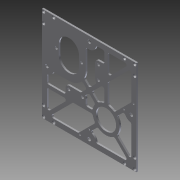
# Autodesk Inventor part: upper gearbox top plate2
Saved by Autodesk Inventor 2012 (Build 160160000, 160)
## iProperties
Created: 2012-07-07
Part Number: upper gearbox top plate2
Material: Default
Document SubType Name: Modeling
Designer: Bryce
Density: 1 g/cm^3
Author: Bryce
Autodesk Inventor part; units mm, degrees
ref_plane "YZ Plane" through (0, 0, 0) normal (1, 0, 0) x (0, 1, 0)
ref_plane "XZ Plane" through (0, 0, 0) normal (0, 1, 0) x (-1, 0, 0)
ref_plane "XY Plane" through (0, 0, 0) normal (0, 0, 1) x (1, 0, 0)
sketch "Sketch1" plane through (0, 0, 0) normal (0, 0, 1) x (1, 0, 0)
  line L0 (-114.3, 114.3) -> (63.5, 114.3)
  line L1 (63.5, 114.3) -> (63.5, -28.575)
  line L2 (63.5, -63.5) -> (28.575, -63.5)
  line L3 (-114.3, -63.5) -> (-114.3, 114.3)
  circle A0 centre (6.35, -6.35) radius 19.05
  circle A1 centre (41.275, 111.125) radius 1.5875
  circle A2 centre (-92.075, -60.325) radius 1.5875
  circle A3 centre (-111.125, 92.075) radius 1.5875
  circle A4 centre (-111.125, 111.125) radius 1.5875
  circle A5 centre (-92.075, 111.125) radius 1.5875
  circle A6 centre (60.325, 92.075) radius 1.5875
  circle A7 centre (-111.125, -60.325) radius 1.5875
  circle A8 centre (-111.125, -41.275) radius 1.5875
  circle A9 centre (60.325, 111.125) radius 1.5875
  circle A10 centre (-63.5, 73.025) radius 19.05
  circle A11 centre (-63.5, 53.975) radius 19.05
  line L4 (-82.55, 73.025) -> (-44.45, 73.025)
  line L5 (-44.45, 73.025) -> (-44.45, 53.975)
  line L6 (-44.45, 53.975) -> (-82.55, 53.975)
  line L7 (-82.55, 53.975) -> (-82.55, 73.025)
  arc A12 (-13.7147, 9.2246) -> (-18.8508, -3.175) centre (6.35, -6.35) ccw
  arc A13 (26.4147, -21.9246) -> (26.4147, 9.2246) centre (6.35, -6.35) ccw
  arc A14 (-9.2246, -26.4147) -> (21.9246, -26.4147) centre (6.35, -6.35) ccw
  arc A15 (21.9246, 13.7147) -> (9.525, 18.8508) centre (6.35, -6.35) ccw
  line L8 (-63.5, 14.3002) -> (-38.1, 14.3002)
  line L9 (-14.3002, 50.8) -> (-14.3002, 76.2)
  arc A16 (-63.3483, 22.2254) -> (-38.6735, 34.1834) centre (-63.5, 53.975) ccw
  line L10 (53.975, 104.775) -> (53.975, 45.7651)
  line L11 (53.975, -53.975) -> (49.4849, -53.975) construction
  line L12 (-104.775, -53.975) -> (-104.775, 12.7)
  line L13 (-63.3483, 22.2254) -> (-92.4782, 22.2254)
  line L14 (21.9246, -26.4147) -> (36.7849, -41.275)
  line L15 (26.4147, -21.9246) -> (41.275, -36.7849)
  line L16 (-13.7147, -21.9246) -> (-45.7651, -53.975)
  line L17 (-9.2246, -26.4147) -> (-24.1468, -41.337)
  line L18 (-13.7147, 9.2246) -> (-25.4, 20.9099)
  line L19 (-9.2246, 13.7147) -> (-20.9099, 25.4)
  line L20 (26.4147, 9.2246) -> (41.337, 24.1468)
  line L21 (21.9246, 13.7147) -> (53.975, 45.7651)
  arc A17 (-35.1635, 39.6536) -> (-31.75, 53.975) centre (-63.5, 53.975) ccw
  line L22 (53.975, -49.4849) -> (53.975, -53.975) construction
  line L23 (49.4849, -53.975) -> (36.7849, -53.975)
  line L24 (-45.7651, -53.975) -> (-104.775, -53.975)
  arc A18 (-31.75, 7.9502) -> (-33.7416, 12.5683) centre (-38.1, 7.9502) ccw
  line L25 (-104.775, -53.975) -> (-60.325, -9.525)
  line L26 (-104.775, -49.4849) -> (-64.8151, -9.525)
  line L27 (53.975, 104.775) -> (9.525, 60.325)
  line L28 (53.975, 100.2849) -> (9.525, 55.8349)
  line L29 (49.4849, 104.775) -> (9.525, 64.8151)
  line L30 (-40.9899, 14.3002) -> (-29.8901, 25.4)
  line L31 (-20.9099, 25.4) -> (-1.8599, 44.45)
  line L32 (-29.8901, 25.4) -> (-38.6735, 34.1834)
  line L33 (-25.4, 29.8901) -> (-35.1635, 39.6536)
  line L34 (-18.8508, -3.175) -> (-31.75, -3.175)
  line L35 (-104.775, -9.525) -> (-64.8151, -9.525)
  line L36 (-69.85, 7.9502) -> (-69.85, -3.175)
  line L37 (-31.75, 7.9502) -> (-31.75, -3.175)
  line L38 (-69.85, -3.175) -> (-104.775, -3.175)
  arc A19 (-31.75, 7.9502) -> (-33.7416, 12.5683) centre (-38.1, 7.9502) ccw
  arc A20 (-18.8508, -9.525) -> (-13.7147, -21.9246) centre (6.35, -6.35) ccw
  line L39 (-55.8349, -9.525) -> (-100.2849, -53.975)
  line L40 (9.525, 104.775) -> (9.525, 64.8151)
  line L41 (3.175, 104.775) -> (3.175, 82.55)
  arc A21 (3.175, 18.8508) -> (-9.2246, 13.7147) centre (6.35, -6.35) ccw
  line L42 (-7.9502, 82.55) -> (3.175, 82.55)
  line L43 (-7.9502, 44.45) -> (3.175, 44.45)
  line L44 (3.175, 44.45) -> (3.175, 18.8508)
  line L45 (-55.8349, -9.525) -> (-18.8508, -9.525)
  line L46 (9.525, 55.8349) -> (9.525, 18.8508)
  arc A22 (-33.7416, 12.5683) -> (-38.1, 14.3002) centre (-38.1, 7.9502) ccw
  arc A23 (-33.7416, 12.5683) -> (-38.1, 14.3002) centre (-38.1, 7.9502) ccw
  line L47 (-33.7416, 12.5683) -> (-25.4, 20.9099)
  arc A24 (-63.5, 14.3002) -> (-69.85, 7.9502) centre (-63.5, 7.9502) ccw
  line L48 (36.7849, -53.975) -> (-12.7, -53.975)
  line L49 (53.975, -36.7849) -> (53.975, -49.4849)
  line L50 (41.275, -36.7849) -> (53.975, -49.4849)
  line L51 (36.7849, -41.275) -> (49.4849, -53.975)
  line L52 (28.575, -63.5) -> (-114.3, -63.5)
  line L53 (63.5, -28.575) -> (63.5, -63.5)
  line L54 (-25.4, -53.975) -> (-25.4, -63.5) construction
  circle A25 centre (41.275, -60.325) radius 1.5875
  circle A26 centre (60.325, -60.325) radius 1.5875
  circle A27 centre (60.325, -41.275) radius 1.5875
  arc A28 (-7.9502, 82.55) -> (-14.3002, 76.2) centre (-7.9502, 76.2) ccw
  line L55 (6.35, -6.35) -> (-25.0809, -37.7809) construction
  line L56 (-43.0414, -55.7414) -> (-50.8, -63.5) construction
  line L57 (-25.0809, -37.7809) -> (-43.0414, -55.7414) construction
  line L58 (6.35, -6.35) -> (40.026, 27.326) construction
  line L59 (40.026, 27.326) -> (57.9865, 45.2865) construction
  line L60 (57.9865, 45.2865) -> (63.5, 50.8) construction
  arc A29 (-12.7, -53.975) -> (-24.1468, -41.337) centre (-25.4, -53.975) ccw
  arc A30 (41.337, 24.1468) -> (53.975, 12.7) centre (53.975, 25.4) ccw
  line L61 (53.975, 12.7) -> (53.975, -36.7849)
  arc A31 (-31.75, 93.7765) -> (-12.7, 104.775) centre (-25.4, 104.775) ccw
  line L62 (-31.75, 93.7765) -> (-31.75, 53.975)
  line L63 (-12.7, 104.775) -> (53.975, 104.775)
  arc A32 (-104.775, 12.7) -> (-92.4782, 22.2254) centre (-104.775, 25.4) ccw
  arc A33 (-14.3002, 50.8) -> (-7.9502, 44.45) centre (-7.9502, 50.8) ccw
  line L64 (-25.4, 29.8901) -> (-10.3636, 44.9265)
  point P0 (0, 0)
  point P1 (-87.3125, 63.5)
  point P2 (-39.6875, 63.5)
  point P3 (-38.1, 7.9502)
  dimension "d87" = 38.1
  dimension "d89" = 38.1
  dimension "d0" = 114.3
  dimension "d1" = 177.8
  dimension "d2" = 177.8
  dimension "d3" = 114.3
  dimension "d4" = 38.1
  dimension "d5" = 57.15
  dimension "d6" = 57.15
  dimension "d10" = 3.175
  dimension "d12" = 3.175
  dimension "d15" = 3.175
  dimension "d16" = 22.225
  dimension "d19" = 3.175
  dimension "d20" = 22.225
  dimension "d23" = 3.175
  dimension "d24" = 3.175
  dimension "d25" = 22.225
  dimension "d26" = 3.175
  dimension "d27" = 3.175
  dimension "d28" = 3.175
  dimension "d29" = 3.175
  dimension "d30" = 22.225
  dimension "d34" = 3.175
  dimension "d35" = 3.175
  dimension "d36" = 3.175
  dimension "d37" = 3.175
  dimension "d38" = 22.225
  dimension "d39" = 3.175
  dimension "d40" = 3.175
  dimension "d47" = 3.175
  dimension "d48" = 3.175
  dimension "d49" = 3.175
  dimension "d50" = 3.175
  dimension "d51" = 22.225
  dimension "d52" = 3.175
  dimension "d88" = 41.275
  dimension "d91" = 50.8
  dimension "d95" = 19.05
  dimension "d98" = 23.8125
  dimension "d99" = 23.8125
  dimension "d112" = 25.4
  dimension "d113" = 71.4502
  dimension "d114" = 50.8
  dimension "d122" = 71.4502
  dimension "d123" = 25.4
  dimension "d124" = 38.1
  dimension "d140" = 25.4
  dimension "d141" = 25.4
  dimension "d142" = 25.4
  dimension "d143" = 25.4
  dimension "d160" = 6.35
  dimension "d163" = 6.35
  dimension "d167" = 9.525
  dimension "d168" = 9.525
  dimension "d169" = 31.75
  dimension "d171" = 158.75
  dimension "d172" = 158.75
  dimension "d173" = 9.525
  dimension "d174" = 9.525
  dimension "d177" = 92.0746
  dimension "d180" = 45
  dimension "d182" = 6.35
  dimension "d183" = 6.35
  dimension "d186" = 6.35
  dimension "d188" = 6.35
  constraints: 131 end point, 43 point on circle, 41 parallel, 32 centre point, 28 perpendicular, 26 point on line, 13 coincident, 12 collinear, 8 tangent, 5 horizontal alignment, 4 horizontal, 4 vertical alignment, 3 symmetric about line, 2 midpoint, 7 other
  measures "d0" distance from line of L0 point (0, 0)
  measures "d1" distance of L0.end L2.start
  measures "d2" distance of L0.start L0.end
  measures "d3" distance from line of L3 point (0, 0)
  measures "d4" diameter of A0
  measures "d5" distance from line of L1 A0.centre
  measures "d6" distance from line of L2 A0.centre
  measures "d10" diameter of A1
  measures "d12" diameter of A2
  measures "d15" distance from line of L0 A1.centre
  measures "d16" distance from line of L1 A1.centre
  measures "d19" distance from line of L2 A2.centre
  measures "d20" distance from line of L3 A2.centre
  measures "d23" diameter of A3
  measures "d24" distance from line of L3 A3.centre
  measures "d25" distance from line of L0 A3.centre
  measures "d26" diameter of A4
  measures "d27" distance from line of L0 A4.centre
  measures "d28" distance from line of L3 A4.centre
  measures "d29" distance from line of L0 A5.centre
  measures "d30" distance from line of L3 A5.centre
  measures "d34" diameter of A9
  measures "d35" distance from line of L0 A9.centre
  measures "d36" distance from line of L1 A9.centre
  measures "d37" distance from line of L1 A6.centre
  measures "d38" distance from line of L0 A6.centre
  measures "d39" diameter of A6
  measures "d40" diameter of A5
  measures "d47" diameter of A7
  measures "d48" distance from line of L2 A7.centre
  measures "d49" distance from line of L3 A7.centre
  measures "d50" diameter of A8
  measures "d51" distance from line of L2 A8.centre
  measures "d52" distance from line of L3 A8.centre
  measures "d88" distance from line of L0 point (-63.5, 73.025)
  measures "d91" distance from line of point (-63.5, 53.975) L3
  measures "d95" distance of L6.end L4.start
  measures "d98" horizontal distance of point (-63.5, 53.975) point (-87.313, 63.5)
  measures "d99" horizontal distance of point (-39.688, 63.5) point (-63.5, 73.025)
  measures "d112" distance of point (-38.1, 7.95) point (-63.5, 7.95)
  measures "d113" distance from line of L2 point (-38.1, 7.95)
  measures "d114" distance from line of L3 point (-63.5, 7.95)
  measures "d122" distance from line of L1 point (-7.95, 76.2)
  measures "d123" distance of point (-7.95, 50.8) point (-7.95, 76.2)
  measures "d124" distance from line of L0 point (-7.95, 76.2)
  measures "d140" radius of A13
  measures "d141" radius of A14
  measures "d142" radius of A12
  measures "d143" radius of A15
  measures "d160" distance from line of point (-63.5, 7.95) L8
  measures "d163" distance from line of L9 point (-7.95, 50.8)
  measures "d167" distance from line of L4 point (-87.313, 63.5)
  measures "d168" distance from line of L4 point (-39.688, 63.5)
  measures "d169" radius of A16
  measures "d171" distance of L11.start L12.start
  measures "d172" distance of L10.start L11.start
  measures "d173" distance between parallel lines of L2 L11
  measures "d174" distance between parallel lines of L1 L10
  measures "d177" distance between parallel lines of L0 L13
  measures "d180" angle of L11 L14
  measures "d182" distance between parallel lines of L15 L14
  measures "d183" distance between parallel lines of L16 L17
  measures "d186" distance between parallel lines of L19 L18
  measures "d188" distance between parallel lines of L21 L20
extrude "Extrusion8" add sketch "Sketch1" along normal blind 3.175
fillet "Fillet3" radius 3.175 41 edges at (21.9246, -26.4147, 1.5875) (49.4849, -53.975, 1.5875) (53.975, -49.4849, 1.5875) (-9.2246, -26.4147, 1.5875) (26.4147, 9.2246, 1.5875) (26.4147, -21.9246, 1.5875) (-18.8508, -9.525, 1.5875) (9.525, 18.8508, 1.5875) (21.9246, 13.7147, 1.5875) (-13.7147, -21.9246, 1.5875) (-45.7651, -53.975, 1.5875) (53.975, 45.7651, 1.5875) (-55.8349, -9.525, 1.5875) (-100.2849, -53.975, 1.5875) (53.975, 100.2849, 1.5875) (9.525, 55.8349, 1.5875) (-18.8508, -3.175, 1.5875) (-31.75, -3.175, 1.5875) (3.175, 44.45, 1.5875) (3.175, 18.8508, 1.5875) (-9.2246, 13.7147, 1.5875) (-20.9099, 25.4, 1.5875) (-1.8599, 44.45, 1.5875) (-33.7416, 12.5683, 1.5875) (-25.4, 20.9099, 1.5875) (-13.7147, 9.2246, 1.5875) (-104.775, -9.525, 1.5875) (-104.775, -49.4849, 1.5875) (-64.8151, -9.525, 1.5875) (9.525, 64.8151, 1.5875) (49.4849, 104.775, 1.5875) (9.525, 104.775, 1.5875) (-104.775, -3.175, 1.5875) (-69.85, -3.175, 1.5875) (-40.9899, 14.3002, 1.5875) (-29.8901, 25.4, 1.5875) (-38.6735, 34.1834, 1.5875) (-25.4, 29.8901, 1.5875) (3.175, 82.55, 1.5875) (3.175, 104.775, 1.5875) (-35.1635, 39.6536, 1.5875)
hole "Hole5" at (-87.3125, 63.5, 0) at (-39.6875, 63.5, 0) at (-63.5, 7.9502, 0) at (-38.1, 7.9502, 0) at (-7.9502, 50.8, 0) at (-7.9502, 76.2, 0) direction (0, 0, 1) diameter 5.08 end through all
hole "Hole6" at (-43.0414, -55.7414, 0) at (-25.0809, -37.7809, 0) direction (0, 0, 1) diameter 3.175 end through all
hole "Hole7" at (40.026, 27.326, 0) at (57.9865, 45.2865, 0) direction (0, 0, 1) diameter 3.175 end through all
chamfer "Chamfer1" distance 1.5875 angle 45 12 edges at (-112.7125, -60.325, 3.175) (-112.7125, -41.275, 3.175) (-93.6625, -60.325, 3.175) (39.6875, -60.325, 3.175) (58.7375, -60.325, 3.175) (58.7375, -41.275, 3.175) (58.7375, 92.075, 3.175) (58.7375, 111.125, 3.175) (39.6875, 111.125, 3.175) (-93.6625, 111.125, 3.175) (-112.7125, 111.125, 3.175) (-112.7125, 92.075, 3.175)
hole "Hole8" at (-25.4, -53.975, 0) at (53.975, 25.4, 0) at (-25.4, 104.775, 0) at (-104.775, 25.4, 0) direction (0, 0, 1) diameter 6.35 end through all
fillet "Fillet4" radius 3.175 8 edges at (-92.4782, 22.2254, 1.5875) (-104.775, 12.7, 1.5875) (-24.1468, -41.337, 1.5875) (-12.7, -53.975, 1.5875) (53.975, 12.7, 1.5875) (41.337, 24.1468, 1.5875) (-12.7, 104.775, 1.5875) (-31.75, 93.7765, 1.5875)
fillet "Fillet5" radius 3.175 1 edges at (-10.3636, 44.9265, 1.5875)
equation "\"d89\" = d87"
body "Solid5"
